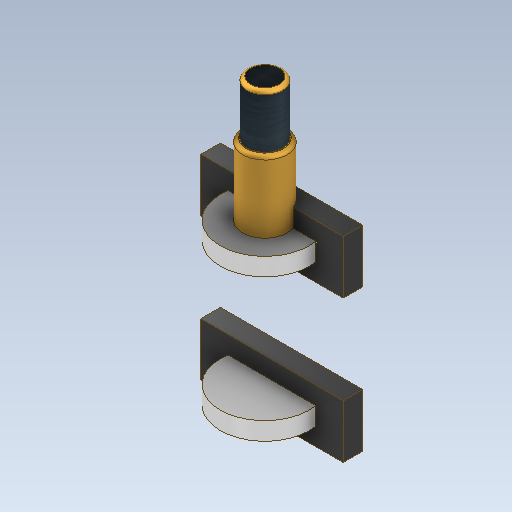
# Autodesk Inventor part: joint 2
Saved by Autodesk Inventor 2020 (Build 240168000, 168)
## iProperties
Created: 2020-07-11
Part Number: joint 2
Material: Aluminum 6061
Document SubType Name: Modeling
Designer: Vikki
Mass: 269.594 g
Surface Area: 274.025 cm^2
Volume: 99.8495 cm^3
Density: 2.7 g/cm^3
Appearance: Brass - Satin
Author: Vikki
Autodesk Inventor part; units mm, degrees
ref_plane "YZ Plane" through (0, 0, 0) normal (1, 0, 0) x (0, 1, 0)
ref_plane "XZ Plane" through (0, 0, 0) normal (0, 1, 0) x (-1, 0, 0)
ref_plane "XY Plane" through (0, 0, 0) normal (0, 0, 1) x (1, 0, 0)
ref_plane "Work Plane1" through (-25, -80, 5) normal (0, -1, 0) x (1, 0, 0)
ref_plane "Work Plane2" through (0, 0, 0) normal (0, 0, 1) x (1, 0, 0)
sketch "Sketch1" plane through (0, 0, 0) normal (0, 0, 1) x (1, 0, 0)
  line L0 (-65, -15) -> (15, -15)
  line L1 (15, -15) -> (15, 15)
  line L2 (15, 15) -> (-65, 15)
  line L3 (-65, 15) -> (-65, -15)
  line L4 (-65, -95) -> (15, -95)
  line L5 (15, -95) -> (15, -65)
  line L6 (15, -65) -> (-65, -65)
  line L7 (-65, -65) -> (-65, -95)
  line L8 (-46.7, 10) -> (-41.5, 10) projected
  arc A0 (-46.7, 10) -> (-46.9, 9.8) centre (-46.7, 9.8) ccw projected
  line L9 (-46.9, 8.2) -> (-46.9, 9.8) projected
  arc A1 (-46.9, 8.2) -> (-46.7, 8) centre (-46.7, 8.2) ccw projected
  line L10 (-43.8971, 8) -> (-46.7, 8) projected
  arc A2 (-43.7556, 7.6586) -> (-43.8971, 8) centre (-43.8971, 7.8) ccw projected
  line L11 (-47.3556, 4.0586) -> (-43.7556, 7.6586) projected
  arc A3 (-47.4971, 4) -> (-47.3556, 4.0586) centre (-47.4971, 4.2) ccw projected
  line L12 (-52.5029, 4) -> (-47.4971, 4) projected
  arc A4 (-52.6444, 4.0586) -> (-52.5029, 4) centre (-52.5029, 4.2) ccw projected
  line L13 (-56.2444, 7.6586) -> (-52.6444, 4.0586) projected
  arc A5 (-56.1029, 8) -> (-56.2444, 7.6586) centre (-56.1029, 7.8) ccw projected
  line L14 (-53.3, 8) -> (-56.1029, 8) projected
  arc A6 (-53.3, 8) -> (-53.1, 8.2) centre (-53.3, 8.2) ccw projected
  line L15 (-53.1, 9.8) -> (-53.1, 8.2) projected
  arc A7 (-53.1, 9.8) -> (-53.3, 10) centre (-53.3, 9.8) ccw projected
  line L16 (-58.5, 10) -> (-53.3, 10) projected
  arc A8 (-58.5, 10) -> (-60, 8.5) centre (-58.5, 8.5) ccw projected
  line L17 (-60, 3.3) -> (-60, 8.5) projected
  arc A9 (-60, 3.3) -> (-59.8, 3.1) centre (-59.8, 3.3) ccw projected
  line L18 (-58.2, 3.1) -> (-59.8, 3.1) projected
  arc A10 (-58.2, 3.1) -> (-58, 3.3) centre (-58.2, 3.3) ccw projected
  line L19 (-58, 6.1029) -> (-58, 3.3) projected
  arc A11 (-57.6586, 6.2444) -> (-58, 6.1029) centre (-57.8, 6.1029) ccw projected
  line L20 (-54.0586, 2.6444) -> (-57.6586, 6.2444) projected
  arc A12 (-54, 2.5029) -> (-54.0586, 2.6444) centre (-54.2, 2.5029) ccw projected
  line L21 (-54, -2.5029) -> (-54, 2.5029) projected
  arc A13 (-54.0586, -2.6444) -> (-54, -2.5029) centre (-54.2, -2.5029) ccw projected
  line L22 (-57.6586, -6.2444) -> (-54.0586, -2.6444) projected
  arc A14 (-58, -6.1029) -> (-57.6586, -6.2444) centre (-57.8, -6.1029) ccw projected
  line L23 (-58, -3.3) -> (-58, -6.1029) projected
  arc A15 (-58, -3.3) -> (-58.2, -3.1) centre (-58.2, -3.3) ccw projected
  line L24 (-59.8, -3.1) -> (-58.2, -3.1) projected
  arc A16 (-59.8, -3.1) -> (-60, -3.3) centre (-59.8, -3.3) ccw projected
  line L25 (-60, -8.5) -> (-60, -3.3) projected
  arc A17 (-60, -8.5) -> (-58.5, -10) centre (-58.5, -8.5) ccw projected
  line L26 (-53.3, -10) -> (-58.5, -10) projected
  arc A18 (-53.3, -10) -> (-53.1, -9.8) centre (-53.3, -9.8) ccw projected
  line L27 (-53.1, -8.2) -> (-53.1, -9.8) projected
  arc A19 (-53.1, -8.2) -> (-53.3, -8) centre (-53.3, -8.2) ccw projected
  line L28 (-56.1029, -8) -> (-53.3, -8) projected
  arc A20 (-56.2444, -7.6586) -> (-56.1029, -8) centre (-56.1029, -7.8) ccw projected
  line L29 (-52.6444, -4.0586) -> (-56.2444, -7.6586) projected
  arc A21 (-52.5029, -4) -> (-52.6444, -4.0586) centre (-52.5029, -4.2) ccw projected
  line L30 (-47.4971, -4) -> (-52.5029, -4) projected
  arc A22 (-47.3556, -4.0586) -> (-47.4971, -4) centre (-47.4971, -4.2) ccw projected
  line L31 (-43.7556, -7.6586) -> (-47.3556, -4.0586) projected
  arc A23 (-43.8971, -8) -> (-43.7556, -7.6586) centre (-43.8971, -7.8) ccw projected
  line L32 (-46.7, -8) -> (-43.8971, -8) projected
  arc A24 (-46.7, -8) -> (-46.9, -8.2) centre (-46.7, -8.2) ccw projected
  line L33 (-46.9, -9.8) -> (-46.9, -8.2) projected
  arc A25 (-46.9, -9.8) -> (-46.7, -10) centre (-46.7, -9.8) ccw projected
  line L34 (-41.5, -10) -> (-46.7, -10) projected
  arc A26 (-41.5, -10) -> (-40, -8.5) centre (-41.5, -8.5) ccw projected
  line L35 (-40, -3.3) -> (-40, -8.5) projected
  arc A27 (-40, -3.3) -> (-40.2, -3.1) centre (-40.2, -3.3) ccw projected
  line L36 (-41.8, -3.1) -> (-40.2, -3.1) projected
  arc A28 (-41.8, -3.1) -> (-42, -3.3) centre (-41.8, -3.3) ccw projected
  line L37 (-42, -6.1029) -> (-42, -3.3) projected
  arc A29 (-42.3414, -6.2444) -> (-42, -6.1029) centre (-42.2, -6.1029) ccw projected
  line L38 (-45.9414, -2.6444) -> (-42.3414, -6.2444) projected
  arc A30 (-46, -2.5029) -> (-45.9414, -2.6444) centre (-45.8, -2.5029) ccw projected
  line L39 (-46, 2.5029) -> (-46, -2.5029) projected
  arc A31 (-45.9414, 2.6444) -> (-46, 2.5029) centre (-45.8, 2.5029) ccw projected
  line L40 (-42.3414, 6.2444) -> (-45.9414, 2.6444) projected
  arc A32 (-42, 6.1029) -> (-42.3414, 6.2444) centre (-42.2, 6.1029) ccw projected
  line L41 (-42, 3.3) -> (-42, 6.1029) projected
  arc A33 (-42, 3.3) -> (-41.8, 3.1) centre (-41.8, 3.3) ccw projected
  line L42 (-40.2, 3.1) -> (-41.8, 3.1) projected
  arc A34 (-40.2, 3.1) -> (-40, 3.3) centre (-40.2, 3.3) ccw projected
  line L43 (-40, 8.5) -> (-40, 3.3) projected
  arc A35 (-40, 8.5) -> (-41.5, 10) centre (-41.5, 8.5) ccw projected
  circle A36 centre (-50, 0) radius 2 projected
  line L44 (3.3, 10) -> (8.5, 10) projected
  arc A37 (3.3, 10) -> (3.1, 9.8) centre (3.3, 9.8) ccw projected
  line L45 (3.1, 8.2) -> (3.1, 9.8) projected
  arc A38 (3.1, 8.2) -> (3.3, 8) centre (3.3, 8.2) ccw projected
  line L46 (6.1029, 8) -> (3.3, 8) projected
  arc A39 (6.2444, 7.6586) -> (6.1029, 8) centre (6.1029, 7.8) ccw projected
  line L47 (2.6444, 4.0586) -> (6.2444, 7.6586) projected
  arc A40 (2.5029, 4) -> (2.6444, 4.0586) centre (2.5029, 4.2) ccw projected
  line L48 (-2.5029, 4) -> (2.5029, 4) projected
  arc A41 (-2.6444, 4.0586) -> (-2.5029, 4) centre (-2.5029, 4.2) ccw projected
  line L49 (-6.2444, 7.6586) -> (-2.6444, 4.0586) projected
  arc A42 (-6.1029, 8) -> (-6.2444, 7.6586) centre (-6.1029, 7.8) ccw projected
  line L50 (-3.3, 8) -> (-6.1029, 8) projected
  arc A43 (-3.3, 8) -> (-3.1, 8.2) centre (-3.3, 8.2) ccw projected
  line L51 (-3.1, 9.8) -> (-3.1, 8.2) projected
  arc A44 (-3.1, 9.8) -> (-3.3, 10) centre (-3.3, 9.8) ccw projected
  line L52 (-8.5, 10) -> (-3.3, 10) projected
  arc A45 (-8.5, 10) -> (-10, 8.5) centre (-8.5, 8.5) ccw projected
  line L53 (-10, 3.3) -> (-10, 8.5) projected
  arc A46 (-10, 3.3) -> (-9.8, 3.1) centre (-9.8, 3.3) ccw projected
  line L54 (-8.2, 3.1) -> (-9.8, 3.1) projected
  arc A47 (-8.2, 3.1) -> (-8, 3.3) centre (-8.2, 3.3) ccw projected
  line L55 (-8, 6.1029) -> (-8, 3.3) projected
  arc A48 (-7.6586, 6.2444) -> (-8, 6.1029) centre (-7.8, 6.1029) ccw projected
  line L56 (-4.0586, 2.6444) -> (-7.6586, 6.2444) projected
  arc A49 (-4, 2.5029) -> (-4.0586, 2.6444) centre (-4.2, 2.5029) ccw projected
  line L57 (-4, -2.5029) -> (-4, 2.5029) projected
  arc A50 (-4.0586, -2.6444) -> (-4, -2.5029) centre (-4.2, -2.5029) ccw projected
  line L58 (-7.6586, -6.2444) -> (-4.0586, -2.6444) projected
  arc A51 (-8, -6.1029) -> (-7.6586, -6.2444) centre (-7.8, -6.1029) ccw projected
  line L59 (-8, -3.3) -> (-8, -6.1029) projected
  arc A52 (-8, -3.3) -> (-8.2, -3.1) centre (-8.2, -3.3) ccw projected
  line L60 (-9.8, -3.1) -> (-8.2, -3.1) projected
  arc A53 (-9.8, -3.1) -> (-10, -3.3) centre (-9.8, -3.3) ccw projected
  line L61 (-10, -8.5) -> (-10, -3.3) projected
  arc A54 (-10, -8.5) -> (-8.5, -10) centre (-8.5, -8.5) ccw projected
  line L62 (-3.3, -10) -> (-8.5, -10) projected
  arc A55 (-3.3, -10) -> (-3.1, -9.8) centre (-3.3, -9.8) ccw projected
  line L63 (-3.1, -8.2) -> (-3.1, -9.8) projected
  arc A56 (-3.1, -8.2) -> (-3.3, -8) centre (-3.3, -8.2) ccw projected
  line L64 (-6.1029, -8) -> (-3.3, -8) projected
  arc A57 (-6.2444, -7.6586) -> (-6.1029, -8) centre (-6.1029, -7.8) ccw projected
  line L65 (-2.6444, -4.0586) -> (-6.2444, -7.6586) projected
  arc A58 (-2.5029, -4) -> (-2.6444, -4.0586) centre (-2.5029, -4.2) ccw projected
  line L66 (2.5029, -4) -> (-2.5029, -4) projected
  arc A59 (2.6444, -4.0586) -> (2.5029, -4) centre (2.5029, -4.2) ccw projected
  line L67 (6.2444, -7.6586) -> (2.6444, -4.0586) projected
  arc A60 (6.1029, -8) -> (6.2444, -7.6586) centre (6.1029, -7.8) ccw projected
  line L68 (3.3, -8) -> (6.1029, -8) projected
  arc A61 (3.3, -8) -> (3.1, -8.2) centre (3.3, -8.2) ccw projected
  line L69 (3.1, -9.8) -> (3.1, -8.2) projected
  arc A62 (3.1, -9.8) -> (3.3, -10) centre (3.3, -9.8) ccw projected
  line L70 (8.5, -10) -> (3.3, -10) projected
  arc A63 (8.5, -10) -> (10, -8.5) centre (8.5, -8.5) ccw projected
  line L71 (10, -3.3) -> (10, -8.5) projected
  arc A64 (10, -3.3) -> (9.8, -3.1) centre (9.8, -3.3) ccw projected
  line L72 (8.2, -3.1) -> (9.8, -3.1) projected
  arc A65 (8.2, -3.1) -> (8, -3.3) centre (8.2, -3.3) ccw projected
  line L73 (8, -6.1029) -> (8, -3.3) projected
  arc A66 (7.6586, -6.2444) -> (8, -6.1029) centre (7.8, -6.1029) ccw projected
  line L74 (4.0586, -2.6444) -> (7.6586, -6.2444) projected
  arc A67 (4, -2.5029) -> (4.0586, -2.6444) centre (4.2, -2.5029) ccw projected
  line L75 (4, 2.5029) -> (4, -2.5029) projected
  arc A68 (4.0586, 2.6444) -> (4, 2.5029) centre (4.2, 2.5029) ccw projected
  line L76 (7.6586, 6.2444) -> (4.0586, 2.6444) projected
  arc A69 (8, 6.1029) -> (7.6586, 6.2444) centre (7.8, 6.1029) ccw projected
  line L77 (8, 3.3) -> (8, 6.1029) projected
  arc A70 (8, 3.3) -> (8.2, 3.1) centre (8.2, 3.3) ccw projected
  line L78 (9.8, 3.1) -> (8.2, 3.1) projected
  arc A71 (9.8, 3.1) -> (10, 3.3) centre (9.8, 3.3) ccw projected
  line L79 (10, 8.5) -> (10, 3.3) projected
  arc A72 (10, 8.5) -> (8.5, 10) centre (8.5, 8.5) ccw projected
  circle A73 centre (0, 0) radius 2 projected
  line L80 (-46.7, -70) -> (-41.5, -70) projected
  arc A74 (-46.7, -70) -> (-46.9, -70.2) centre (-46.7, -70.2) ccw projected
  line L81 (-46.9, -71.8) -> (-46.9, -70.2) projected
  arc A75 (-46.9, -71.8) -> (-46.7, -72) centre (-46.7, -71.8) ccw projected
  line L82 (-43.8971, -72) -> (-46.7, -72) projected
  arc A76 (-43.7556, -72.3414) -> (-43.8971, -72) centre (-43.8971, -72.2) ccw projected
  line L83 (-47.3556, -75.9414) -> (-43.7556, -72.3414) projected
  arc A77 (-47.4971, -76) -> (-47.3556, -75.9414) centre (-47.4971, -75.8) ccw projected
  line L84 (-52.5029, -76) -> (-47.4971, -76) projected
  arc A78 (-52.6444, -75.9414) -> (-52.5029, -76) centre (-52.5029, -75.8) ccw projected
  line L85 (-56.2444, -72.3414) -> (-52.6444, -75.9414) projected
  arc A79 (-56.1029, -72) -> (-56.2444, -72.3414) centre (-56.1029, -72.2) ccw projected
  line L86 (-53.3, -72) -> (-56.1029, -72) projected
  arc A80 (-53.3, -72) -> (-53.1, -71.8) centre (-53.3, -71.8) ccw projected
  line L87 (-53.1, -70.2) -> (-53.1, -71.8) projected
  arc A81 (-53.1, -70.2) -> (-53.3, -70) centre (-53.3, -70.2) ccw projected
  line L88 (-58.5, -70) -> (-53.3, -70) projected
  arc A82 (-58.5, -70) -> (-60, -71.5) centre (-58.5, -71.5) ccw projected
  line L89 (-60, -76.7) -> (-60, -71.5) projected
  arc A83 (-60, -76.7) -> (-59.8, -76.9) centre (-59.8, -76.7) ccw projected
  line L90 (-58.2, -76.9) -> (-59.8, -76.9) projected
  arc A84 (-58.2, -76.9) -> (-58, -76.7) centre (-58.2, -76.7) ccw projected
  line L91 (-58, -73.8971) -> (-58, -76.7) projected
  arc A85 (-57.6586, -73.7556) -> (-58, -73.8971) centre (-57.8, -73.8971) ccw projected
  line L92 (-54.0586, -77.3556) -> (-57.6586, -73.7556) projected
  arc A86 (-54, -77.4971) -> (-54.0586, -77.3556) centre (-54.2, -77.4971) ccw projected
  line L93 (-54, -82.5029) -> (-54, -77.4971) projected
  arc A87 (-54.0586, -82.6444) -> (-54, -82.5029) centre (-54.2, -82.5029) ccw projected
  line L94 (-57.6586, -86.2444) -> (-54.0586, -82.6444) projected
  arc A88 (-58, -86.1029) -> (-57.6586, -86.2444) centre (-57.8, -86.1029) ccw projected
  line L95 (-58, -83.3) -> (-58, -86.1029) projected
  arc A89 (-58, -83.3) -> (-58.2, -83.1) centre (-58.2, -83.3) ccw projected
  line L96 (-59.8, -83.1) -> (-58.2, -83.1) projected
  arc A90 (-59.8, -83.1) -> (-60, -83.3) centre (-59.8, -83.3) ccw projected
  line L97 (-60, -88.5) -> (-60, -83.3) projected
  arc A91 (-60, -88.5) -> (-58.5, -90) centre (-58.5, -88.5) ccw projected
  line L98 (-53.3, -90) -> (-58.5, -90) projected
  arc A92 (-53.3, -90) -> (-53.1, -89.8) centre (-53.3, -89.8) ccw projected
  line L99 (-53.1, -88.2) -> (-53.1, -89.8) projected
  arc A93 (-53.1, -88.2) -> (-53.3, -88) centre (-53.3, -88.2) ccw projected
  line L100 (-56.1029, -88) -> (-53.3, -88) projected
  arc A94 (-56.2444, -87.6586) -> (-56.1029, -88) centre (-56.1029, -87.8) ccw projected
  line L101 (-52.6444, -84.0586) -> (-56.2444, -87.6586) projected
  arc A95 (-52.5029, -84) -> (-52.6444, -84.0586) centre (-52.5029, -84.2) ccw projected
  line L102 (-47.4971, -84) -> (-52.5029, -84) projected
  arc A96 (-47.3556, -84.0586) -> (-47.4971, -84) centre (-47.4971, -84.2) ccw projected
  line L103 (-43.7556, -87.6586) -> (-47.3556, -84.0586) projected
  arc A97 (-43.8971, -88) -> (-43.7556, -87.6586) centre (-43.8971, -87.8) ccw projected
  line L104 (-46.7, -88) -> (-43.8971, -88) projected
  arc A98 (-46.7, -88) -> (-46.9, -88.2) centre (-46.7, -88.2) ccw projected
  line L105 (-46.9, -89.8) -> (-46.9, -88.2) projected
  arc A99 (-46.9, -89.8) -> (-46.7, -90) centre (-46.7, -89.8) ccw projected
  line L106 (-41.5, -90) -> (-46.7, -90) projected
  arc A100 (-41.5, -90) -> (-40, -88.5) centre (-41.5, -88.5) ccw projected
  line L107 (-40, -83.3) -> (-40, -88.5) projected
  arc A101 (-40, -83.3) -> (-40.2, -83.1) centre (-40.2, -83.3) ccw projected
  line L108 (-41.8, -83.1) -> (-40.2, -83.1) projected
  arc A102 (-41.8, -83.1) -> (-42, -83.3) centre (-41.8, -83.3) ccw projected
  line L109 (-42, -86.1029) -> (-42, -83.3) projected
  arc A103 (-42.3414, -86.2444) -> (-42, -86.1029) centre (-42.2, -86.1029) ccw projected
  line L110 (-45.9414, -82.6444) -> (-42.3414, -86.2444) projected
  arc A104 (-46, -82.5029) -> (-45.9414, -82.6444) centre (-45.8, -82.5029) ccw projected
  line L111 (-46, -77.4971) -> (-46, -82.5029) projected
  arc A105 (-45.9414, -77.3556) -> (-46, -77.4971) centre (-45.8, -77.4971) ccw projected
  line L112 (-42.3414, -73.7556) -> (-45.9414, -77.3556) projected
  arc A106 (-42, -73.8971) -> (-42.3414, -73.7556) centre (-42.2, -73.8971) ccw projected
  line L113 (-42, -76.7) -> (-42, -73.8971) projected
  arc A107 (-42, -76.7) -> (-41.8, -76.9) centre (-41.8, -76.7) ccw projected
  line L114 (-40.2, -76.9) -> (-41.8, -76.9) projected
  arc A108 (-40.2, -76.9) -> (-40, -76.7) centre (-40.2, -76.7) ccw projected
  line L115 (-40, -71.5) -> (-40, -76.7) projected
  arc A109 (-40, -71.5) -> (-41.5, -70) centre (-41.5, -71.5) ccw projected
  circle A110 centre (-50, -80) radius 2 projected
  line L116 (3.3, -70) -> (8.5, -70) projected
  arc A111 (3.3, -70) -> (3.1, -70.2) centre (3.3, -70.2) ccw projected
  line L117 (3.1, -71.8) -> (3.1, -70.2) projected
  arc A112 (3.1, -71.8) -> (3.3, -72) centre (3.3, -71.8) ccw projected
  line L118 (6.1029, -72) -> (3.3, -72) projected
  arc A113 (6.2444, -72.3414) -> (6.1029, -72) centre (6.1029, -72.2) ccw projected
  line L119 (2.6444, -75.9414) -> (6.2444, -72.3414) projected
  arc A114 (2.5029, -76) -> (2.6444, -75.9414) centre (2.5029, -75.8) ccw projected
  line L120 (-2.5029, -76) -> (2.5029, -76) projected
  arc A115 (-2.6444, -75.9414) -> (-2.5029, -76) centre (-2.5029, -75.8) ccw projected
  line L121 (-6.2444, -72.3414) -> (-2.6444, -75.9414) projected
  arc A116 (-6.1029, -72) -> (-6.2444, -72.3414) centre (-6.1029, -72.2) ccw projected
  line L122 (-3.3, -72) -> (-6.1029, -72) projected
  arc A117 (-3.3, -72) -> (-3.1, -71.8) centre (-3.3, -71.8) ccw projected
  line L123 (-3.1, -70.2) -> (-3.1, -71.8) projected
  arc A118 (-3.1, -70.2) -> (-3.3, -70) centre (-3.3, -70.2) ccw projected
  line L124 (-8.5, -70) -> (-3.3, -70) projected
  arc A119 (-8.5, -70) -> (-10, -71.5) centre (-8.5, -71.5) ccw projected
  line L125 (-10, -76.7) -> (-10, -71.5) projected
  arc A120 (-10, -76.7) -> (-9.8, -76.9) centre (-9.8, -76.7) ccw projected
  line L126 (-8.2, -76.9) -> (-9.8, -76.9) projected
  arc A121 (-8.2, -76.9) -> (-8, -76.7) centre (-8.2, -76.7) ccw projected
  line L127 (-8, -73.8971) -> (-8, -76.7) projected
  arc A122 (-7.6586, -73.7556) -> (-8, -73.8971) centre (-7.8, -73.8971) ccw projected
  line L128 (-4.0586, -77.3556) -> (-7.6586, -73.7556) projected
  arc A123 (-4, -77.4971) -> (-4.0586, -77.3556) centre (-4.2, -77.4971) ccw projected
  line L129 (-4, -82.5029) -> (-4, -77.4971) projected
  arc A124 (-4.0586, -82.6444) -> (-4, -82.5029) centre (-4.2, -82.5029) ccw projected
  line L130 (-7.6586, -86.2444) -> (-4.0586, -82.6444) projected
  arc A125 (-8, -86.1029) -> (-7.6586, -86.2444) centre (-7.8, -86.1029) ccw projected
  line L131 (-8, -83.3) -> (-8, -86.1029) projected
  arc A126 (-8, -83.3) -> (-8.2, -83.1) centre (-8.2, -83.3) ccw projected
  line L132 (-9.8, -83.1) -> (-8.2, -83.1) projected
  arc A127 (-9.8, -83.1) -> (-10, -83.3) centre (-9.8, -83.3) ccw projected
  line L133 (-10, -88.5) -> (-10, -83.3) projected
  arc A128 (-10, -88.5) -> (-8.5, -90) centre (-8.5, -88.5) ccw projected
  line L134 (-3.3, -90) -> (-8.5, -90) projected
  arc A129 (-3.3, -90) -> (-3.1, -89.8) centre (-3.3, -89.8) ccw projected
  line L135 (-3.1, -88.2) -> (-3.1, -89.8) projected
  arc A130 (-3.1, -88.2) -> (-3.3, -88) centre (-3.3, -88.2) ccw projected
  line L136 (-6.1029, -88) -> (-3.3, -88) projected
  arc A131 (-6.2444, -87.6586) -> (-6.1029, -88) centre (-6.1029, -87.8) ccw projected
  line L137 (-2.6444, -84.0586) -> (-6.2444, -87.6586) projected
  arc A132 (-2.5029, -84) -> (-2.6444, -84.0586) centre (-2.5029, -84.2) ccw projected
  line L138 (2.5029, -84) -> (-2.5029, -84) projected
  arc A133 (2.6444, -84.0586) -> (2.5029, -84) centre (2.5029, -84.2) ccw projected
  line L139 (6.2444, -87.6586) -> (2.6444, -84.0586) projected
  arc A134 (6.1029, -88) -> (6.2444, -87.6586) centre (6.1029, -87.8) ccw projected
  line L140 (3.3, -88) -> (6.1029, -88) projected
  arc A135 (3.3, -88) -> (3.1, -88.2) centre (3.3, -88.2) ccw projected
  line L141 (3.1, -89.8) -> (3.1, -88.2) projected
  arc A136 (3.1, -89.8) -> (3.3, -90) centre (3.3, -89.8) ccw projected
  line L142 (8.5, -90) -> (3.3, -90) projected
  arc A137 (8.5, -90) -> (10, -88.5) centre (8.5, -88.5) ccw projected
  line L143 (10, -83.3) -> (10, -88.5) projected
  arc A138 (10, -83.3) -> (9.8, -83.1) centre (9.8, -83.3) ccw projected
  line L144 (8.2, -83.1) -> (9.8, -83.1) projected
  arc A139 (8.2, -83.1) -> (8, -83.3) centre (8.2, -83.3) ccw projected
  line L145 (8, -86.1029) -> (8, -83.3) projected
  arc A140 (7.6586, -86.2444) -> (8, -86.1029) centre (7.8, -86.1029) ccw projected
  line L146 (4.0586, -82.6444) -> (7.6586, -86.2444) projected
  arc A141 (4, -82.5029) -> (4.0586, -82.6444) centre (4.2, -82.5029) ccw projected
  line L147 (4, -77.4971) -> (4, -82.5029) projected
  arc A142 (4.0586, -77.3556) -> (4, -77.4971) centre (4.2, -77.4971) ccw projected
  line L148 (7.6586, -73.7556) -> (4.0586, -77.3556) projected
  arc A143 (8, -73.8971) -> (7.6586, -73.7556) centre (7.8, -73.8971) ccw projected
  line L149 (8, -76.7) -> (8, -73.8971) projected
  arc A144 (8, -76.7) -> (8.2, -76.9) centre (8.2, -76.7) ccw projected
  line L150 (9.8, -76.9) -> (8.2, -76.9) projected
  arc A145 (9.8, -76.9) -> (10, -76.7) centre (9.8, -76.7) ccw projected
  line L151 (10, -71.5) -> (10, -76.7) projected
  arc A146 (10, -71.5) -> (8.5, -70) centre (8.5, -71.5) ccw projected
  circle A147 centre (0, -80) radius 2 projected
  point P0 (0, 0)
  dimension "d0" = 5
  dimension "d1" = 5
  dimension "d2" = 5
  dimension "d3" = 5
  dimension "d4" = 5
  dimension "d5" = 5
  dimension "d6" = 5
  dimension "d7" = 5
  constraints: 16 end point, 4 parallel, 2 horizontal, 2 perpendicular
  measures "d0" distance between parallel lines of L2 L16
  measures "d1" distance between parallel lines of L0 L34
  measures "d2" distance between parallel lines of L3 L17
  measures "d3" distance between parallel lines of L79 L1
  measures "d4" distance between parallel lines of L7 L89
  measures "d5" distance between parallel lines of L143 L5
  measures "d6" distance between parallel lines of L4 L142
  measures "d7" distance between parallel lines of L6 L124
extrude "Extrusion1" add sketch "Sketch1" against normal blind 10 contours L3 L2 L1 L0 | L7 L6 L5 L4
sketch "Sketch2" plane through (0, 0, 0) normal (0, 0, 1) x (1, 0, 0)
  line L0 (-46.7, -70) -> (-41.5, -70) projected
  arc A0 (-46.7, -70) -> (-46.9, -70.2) centre (-46.7, -70.2) ccw projected
  line L1 (-46.9, -71.8) -> (-46.9, -70.2) projected
  arc A1 (-46.9, -71.8) -> (-46.7, -72) centre (-46.7, -71.8) ccw projected
  line L2 (-43.8971, -72) -> (-46.7, -72) projected
  arc A2 (-43.7556, -72.3414) -> (-43.8971, -72) centre (-43.8971, -72.2) ccw projected
  line L3 (-47.3556, -75.9414) -> (-43.7556, -72.3414) projected
  arc A3 (-47.4971, -76) -> (-47.3556, -75.9414) centre (-47.4971, -75.8) ccw projected
  line L4 (-52.5029, -76) -> (-47.4971, -76) projected
  arc A4 (-52.6444, -75.9414) -> (-52.5029, -76) centre (-52.5029, -75.8) ccw projected
  line L5 (-56.2444, -72.3414) -> (-52.6444, -75.9414) projected
  arc A5 (-56.1029, -72) -> (-56.2444, -72.3414) centre (-56.1029, -72.2) ccw projected
  line L6 (-53.3, -72) -> (-56.1029, -72) projected
  arc A6 (-53.3, -72) -> (-53.1, -71.8) centre (-53.3, -71.8) ccw projected
  line L7 (-53.1, -70.2) -> (-53.1, -71.8) projected
  arc A7 (-53.1, -70.2) -> (-53.3, -70) centre (-53.3, -70.2) ccw projected
  line L8 (-58.5, -70) -> (-53.3, -70) projected
  arc A8 (-58.5, -70) -> (-60, -71.5) centre (-58.5, -71.5) ccw projected
  line L9 (-60, -76.7) -> (-60, -71.5) projected
  arc A9 (-60, -76.7) -> (-59.8, -76.9) centre (-59.8, -76.7) ccw projected
  line L10 (-58.2, -76.9) -> (-59.8, -76.9) projected
  arc A10 (-58.2, -76.9) -> (-58, -76.7) centre (-58.2, -76.7) ccw projected
  line L11 (-58, -73.8971) -> (-58, -76.7) projected
  arc A11 (-57.6586, -73.7556) -> (-58, -73.8971) centre (-57.8, -73.8971) ccw projected
  line L12 (-54.0586, -77.3556) -> (-57.6586, -73.7556) projected
  arc A12 (-54, -77.4971) -> (-54.0586, -77.3556) centre (-54.2, -77.4971) ccw projected
  line L13 (-54, -82.5029) -> (-54, -77.4971) projected
  arc A13 (-54.0586, -82.6444) -> (-54, -82.5029) centre (-54.2, -82.5029) ccw projected
  line L14 (-57.6586, -86.2444) -> (-54.0586, -82.6444) projected
  arc A14 (-58, -86.1029) -> (-57.6586, -86.2444) centre (-57.8, -86.1029) ccw projected
  line L15 (-58, -83.3) -> (-58, -86.1029) projected
  arc A15 (-58, -83.3) -> (-58.2, -83.1) centre (-58.2, -83.3) ccw projected
  line L16 (-59.8, -83.1) -> (-58.2, -83.1) projected
  arc A16 (-59.8, -83.1) -> (-60, -83.3) centre (-59.8, -83.3) ccw projected
  line L17 (-60, -88.5) -> (-60, -83.3) projected
  arc A17 (-60, -88.5) -> (-58.5, -90) centre (-58.5, -88.5) ccw projected
  line L18 (-53.3, -90) -> (-58.5, -90) projected
  arc A18 (-53.3, -90) -> (-53.1, -89.8) centre (-53.3, -89.8) ccw projected
  line L19 (-53.1, -88.2) -> (-53.1, -89.8) projected
  arc A19 (-53.1, -88.2) -> (-53.3, -88) centre (-53.3, -88.2) ccw projected
  line L20 (-56.1029, -88) -> (-53.3, -88) projected
  arc A20 (-56.2444, -87.6586) -> (-56.1029, -88) centre (-56.1029, -87.8) ccw projected
  line L21 (-52.6444, -84.0586) -> (-56.2444, -87.6586) projected
  arc A21 (-52.5029, -84) -> (-52.6444, -84.0586) centre (-52.5029, -84.2) ccw projected
  line L22 (-47.4971, -84) -> (-52.5029, -84) projected
  arc A22 (-47.3556, -84.0586) -> (-47.4971, -84) centre (-47.4971, -84.2) ccw projected
  line L23 (-43.7556, -87.6586) -> (-47.3556, -84.0586) projected
  arc A23 (-43.8971, -88) -> (-43.7556, -87.6586) centre (-43.8971, -87.8) ccw projected
  line L24 (-46.7, -88) -> (-43.8971, -88) projected
  arc A24 (-46.7, -88) -> (-46.9, -88.2) centre (-46.7, -88.2) ccw projected
  line L25 (-46.9, -89.8) -> (-46.9, -88.2) projected
  arc A25 (-46.9, -89.8) -> (-46.7, -90) centre (-46.7, -89.8) ccw projected
  line L26 (-41.5, -90) -> (-46.7, -90) projected
  arc A26 (-41.5, -90) -> (-40, -88.5) centre (-41.5, -88.5) ccw projected
  line L27 (-40, -83.3) -> (-40, -88.5) projected
  arc A27 (-40, -83.3) -> (-40.2, -83.1) centre (-40.2, -83.3) ccw projected
  line L28 (-41.8, -83.1) -> (-40.2, -83.1) projected
  arc A28 (-41.8, -83.1) -> (-42, -83.3) centre (-41.8, -83.3) ccw projected
  line L29 (-42, -86.1029) -> (-42, -83.3) projected
  arc A29 (-42.3414, -86.2444) -> (-42, -86.1029) centre (-42.2, -86.1029) ccw projected
  line L30 (-45.9414, -82.6444) -> (-42.3414, -86.2444) projected
  arc A30 (-46, -82.5029) -> (-45.9414, -82.6444) centre (-45.8, -82.5029) ccw projected
  line L31 (-46, -77.4971) -> (-46, -82.5029) projected
  arc A31 (-45.9414, -77.3556) -> (-46, -77.4971) centre (-45.8, -77.4971) ccw projected
  line L32 (-42.3414, -73.7556) -> (-45.9414, -77.3556) projected
  arc A32 (-42, -73.8971) -> (-42.3414, -73.7556) centre (-42.2, -73.8971) ccw projected
  line L33 (-42, -76.7) -> (-42, -73.8971) projected
  arc A33 (-42, -76.7) -> (-41.8, -76.9) centre (-41.8, -76.7) ccw projected
  line L34 (-40.2, -76.9) -> (-41.8, -76.9) projected
  arc A34 (-40.2, -76.9) -> (-40, -76.7) centre (-40.2, -76.7) ccw projected
  line L35 (-40, -71.5) -> (-40, -76.7) projected
  arc A35 (-40, -71.5) -> (-41.5, -70) centre (-41.5, -71.5) ccw projected
  circle A36 centre (-50, -80) radius 2 projected
  line L36 (3.3, -70) -> (8.5, -70) projected
  arc A37 (3.3, -70) -> (3.1, -70.2) centre (3.3, -70.2) ccw projected
  line L37 (3.1, -71.8) -> (3.1, -70.2) projected
  arc A38 (3.1, -71.8) -> (3.3, -72) centre (3.3, -71.8) ccw projected
  line L38 (6.1029, -72) -> (3.3, -72) projected
  arc A39 (6.2444, -72.3414) -> (6.1029, -72) centre (6.1029, -72.2) ccw projected
  line L39 (2.6444, -75.9414) -> (6.2444, -72.3414) projected
  arc A40 (2.5029, -76) -> (2.6444, -75.9414) centre (2.5029, -75.8) ccw projected
  line L40 (-2.5029, -76) -> (2.5029, -76) projected
  arc A41 (-2.6444, -75.9414) -> (-2.5029, -76) centre (-2.5029, -75.8) ccw projected
  line L41 (-6.2444, -72.3414) -> (-2.6444, -75.9414) projected
  arc A42 (-6.1029, -72) -> (-6.2444, -72.3414) centre (-6.1029, -72.2) ccw projected
  line L42 (-3.3, -72) -> (-6.1029, -72) projected
  arc A43 (-3.3, -72) -> (-3.1, -71.8) centre (-3.3, -71.8) ccw projected
  line L43 (-3.1, -70.2) -> (-3.1, -71.8) projected
  arc A44 (-3.1, -70.2) -> (-3.3, -70) centre (-3.3, -70.2) ccw projected
  line L44 (-8.5, -70) -> (-3.3, -70) projected
  arc A45 (-8.5, -70) -> (-10, -71.5) centre (-8.5, -71.5) ccw projected
  line L45 (-10, -76.7) -> (-10, -71.5) projected
  arc A46 (-10, -76.7) -> (-9.8, -76.9) centre (-9.8, -76.7) ccw projected
  line L46 (-8.2, -76.9) -> (-9.8, -76.9) projected
  arc A47 (-8.2, -76.9) -> (-8, -76.7) centre (-8.2, -76.7) ccw projected
  line L47 (-8, -73.8971) -> (-8, -76.7) projected
  arc A48 (-7.6586, -73.7556) -> (-8, -73.8971) centre (-7.8, -73.8971) ccw projected
  line L48 (-4.0586, -77.3556) -> (-7.6586, -73.7556) projected
  arc A49 (-4, -77.4971) -> (-4.0586, -77.3556) centre (-4.2, -77.4971) ccw projected
  line L49 (-4, -82.5029) -> (-4, -77.4971) projected
  arc A50 (-4.0586, -82.6444) -> (-4, -82.5029) centre (-4.2, -82.5029) ccw projected
  line L50 (-7.6586, -86.2444) -> (-4.0586, -82.6444) projected
  arc A51 (-8, -86.1029) -> (-7.6586, -86.2444) centre (-7.8, -86.1029) ccw projected
  line L51 (-8, -83.3) -> (-8, -86.1029) projected
  arc A52 (-8, -83.3) -> (-8.2, -83.1) centre (-8.2, -83.3) ccw projected
  line L52 (-9.8, -83.1) -> (-8.2, -83.1) projected
  arc A53 (-9.8, -83.1) -> (-10, -83.3) centre (-9.8, -83.3) ccw projected
  line L53 (-10, -88.5) -> (-10, -83.3) projected
  arc A54 (-10, -88.5) -> (-8.5, -90) centre (-8.5, -88.5) ccw projected
  line L54 (-3.3, -90) -> (-8.5, -90) projected
  arc A55 (-3.3, -90) -> (-3.1, -89.8) centre (-3.3, -89.8) ccw projected
  line L55 (-3.1, -88.2) -> (-3.1, -89.8) projected
  arc A56 (-3.1, -88.2) -> (-3.3, -88) centre (-3.3, -88.2) ccw projected
  line L56 (-6.1029, -88) -> (-3.3, -88) projected
  arc A57 (-6.2444, -87.6586) -> (-6.1029, -88) centre (-6.1029, -87.8) ccw projected
  line L57 (-2.6444, -84.0586) -> (-6.2444, -87.6586) projected
  arc A58 (-2.5029, -84) -> (-2.6444, -84.0586) centre (-2.5029, -84.2) ccw projected
  line L58 (2.5029, -84) -> (-2.5029, -84) projected
  arc A59 (2.6444, -84.0586) -> (2.5029, -84) centre (2.5029, -84.2) ccw projected
  line L59 (6.2444, -87.6586) -> (2.6444, -84.0586) projected
  arc A60 (6.1029, -88) -> (6.2444, -87.6586) centre (6.1029, -87.8) ccw projected
  line L60 (3.3, -88) -> (6.1029, -88) projected
  arc A61 (3.3, -88) -> (3.1, -88.2) centre (3.3, -88.2) ccw projected
  line L61 (3.1, -89.8) -> (3.1, -88.2) projected
  arc A62 (3.1, -89.8) -> (3.3, -90) centre (3.3, -89.8) ccw projected
  line L62 (8.5, -90) -> (3.3, -90) projected
  arc A63 (8.5, -90) -> (10, -88.5) centre (8.5, -88.5) ccw projected
  line L63 (10, -83.3) -> (10, -88.5) projected
  arc A64 (10, -83.3) -> (9.8, -83.1) centre (9.8, -83.3) ccw projected
  line L64 (8.2, -83.1) -> (9.8, -83.1) projected
  arc A65 (8.2, -83.1) -> (8, -83.3) centre (8.2, -83.3) ccw projected
  line L65 (8, -86.1029) -> (8, -83.3) projected
  arc A66 (7.6586, -86.2444) -> (8, -86.1029) centre (7.8, -86.1029) ccw projected
  line L66 (4.0586, -82.6444) -> (7.6586, -86.2444) projected
  arc A67 (4, -82.5029) -> (4.0586, -82.6444) centre (4.2, -82.5029) ccw projected
  line L67 (4, -77.4971) -> (4, -82.5029) projected
  arc A68 (4.0586, -77.3556) -> (4, -77.4971) centre (4.2, -77.4971) ccw projected
  line L68 (7.6586, -73.7556) -> (4.0586, -77.3556) projected
  arc A69 (8, -73.8971) -> (7.6586, -73.7556) centre (7.8, -73.8971) ccw projected
  line L69 (8, -76.7) -> (8, -73.8971) projected
  arc A70 (8, -76.7) -> (8.2, -76.9) centre (8.2, -76.7) ccw projected
  line L70 (9.8, -76.9) -> (8.2, -76.9) projected
  arc A71 (9.8, -76.9) -> (10, -76.7) centre (9.8, -76.7) ccw projected
  line L71 (10, -71.5) -> (10, -76.7) projected
  arc A72 (10, -71.5) -> (8.5, -70) centre (8.5, -71.5) ccw projected
  circle A73 centre (0, -80) radius 2 projected
  line L72 (3.3, 10) -> (8.5, 10) projected
  arc A74 (3.3, 10) -> (3.1, 9.8) centre (3.3, 9.8) ccw projected
  line L73 (3.1, 8.2) -> (3.1, 9.8) projected
  arc A75 (3.1, 8.2) -> (3.3, 8) centre (3.3, 8.2) ccw projected
  line L74 (6.1029, 8) -> (3.3, 8) projected
  arc A76 (6.2444, 7.6586) -> (6.1029, 8) centre (6.1029, 7.8) ccw projected
  line L75 (2.6444, 4.0586) -> (6.2444, 7.6586) projected
  arc A77 (2.5029, 4) -> (2.6444, 4.0586) centre (2.5029, 4.2) ccw projected
  line L76 (-2.5029, 4) -> (2.5029, 4) projected
  arc A78 (-2.6444, 4.0586) -> (-2.5029, 4) centre (-2.5029, 4.2) ccw projected
  line L77 (-6.2444, 7.6586) -> (-2.6444, 4.0586) projected
  arc A79 (-6.1029, 8) -> (-6.2444, 7.6586) centre (-6.1029, 7.8) ccw projected
  line L78 (-3.3, 8) -> (-6.1029, 8) projected
  arc A80 (-3.3, 8) -> (-3.1, 8.2) centre (-3.3, 8.2) ccw projected
  line L79 (-3.1, 9.8) -> (-3.1, 8.2) projected
  arc A81 (-3.1, 9.8) -> (-3.3, 10) centre (-3.3, 9.8) ccw projected
  line L80 (-8.5, 10) -> (-3.3, 10) projected
  arc A82 (-8.5, 10) -> (-10, 8.5) centre (-8.5, 8.5) ccw projected
  line L81 (-10, 3.3) -> (-10, 8.5) projected
  arc A83 (-10, 3.3) -> (-9.8, 3.1) centre (-9.8, 3.3) ccw projected
  line L82 (-8.2, 3.1) -> (-9.8, 3.1) projected
  arc A84 (-8.2, 3.1) -> (-8, 3.3) centre (-8.2, 3.3) ccw projected
  line L83 (-8, 6.1029) -> (-8, 3.3) projected
  arc A85 (-7.6586, 6.2444) -> (-8, 6.1029) centre (-7.8, 6.1029) ccw projected
  line L84 (-4.0586, 2.6444) -> (-7.6586, 6.2444) projected
  arc A86 (-4, 2.5029) -> (-4.0586, 2.6444) centre (-4.2, 2.5029) ccw projected
  line L85 (-4, -2.5029) -> (-4, 2.5029) projected
  arc A87 (-4.0586, -2.6444) -> (-4, -2.5029) centre (-4.2, -2.5029) ccw projected
  line L86 (-7.6586, -6.2444) -> (-4.0586, -2.6444) projected
  arc A88 (-8, -6.1029) -> (-7.6586, -6.2444) centre (-7.8, -6.1029) ccw projected
  line L87 (-8, -3.3) -> (-8, -6.1029) projected
  arc A89 (-8, -3.3) -> (-8.2, -3.1) centre (-8.2, -3.3) ccw projected
  line L88 (-9.8, -3.1) -> (-8.2, -3.1) projected
  arc A90 (-9.8, -3.1) -> (-10, -3.3) centre (-9.8, -3.3) ccw projected
  line L89 (-10, -8.5) -> (-10, -3.3) projected
  arc A91 (-10, -8.5) -> (-8.5, -10) centre (-8.5, -8.5) ccw projected
  line L90 (-3.3, -10) -> (-8.5, -10) projected
  arc A92 (-3.3, -10) -> (-3.1, -9.8) centre (-3.3, -9.8) ccw projected
  line L91 (-3.1, -8.2) -> (-3.1, -9.8) projected
  arc A93 (-3.1, -8.2) -> (-3.3, -8) centre (-3.3, -8.2) ccw projected
  line L92 (-6.1029, -8) -> (-3.3, -8) projected
  arc A94 (-6.2444, -7.6586) -> (-6.1029, -8) centre (-6.1029, -7.8) ccw projected
  line L93 (-2.6444, -4.0586) -> (-6.2444, -7.6586) projected
  arc A95 (-2.5029, -4) -> (-2.6444, -4.0586) centre (-2.5029, -4.2) ccw projected
  line L94 (2.5029, -4) -> (-2.5029, -4) projected
  arc A96 (2.6444, -4.0586) -> (2.5029, -4) centre (2.5029, -4.2) ccw projected
  line L95 (6.2444, -7.6586) -> (2.6444, -4.0586) projected
  arc A97 (6.1029, -8) -> (6.2444, -7.6586) centre (6.1029, -7.8) ccw projected
  line L96 (3.3, -8) -> (6.1029, -8) projected
  arc A98 (3.3, -8) -> (3.1, -8.2) centre (3.3, -8.2) ccw projected
  line L97 (3.1, -9.8) -> (3.1, -8.2) projected
  arc A99 (3.1, -9.8) -> (3.3, -10) centre (3.3, -9.8) ccw projected
  line L98 (8.5, -10) -> (3.3, -10) projected
  arc A100 (8.5, -10) -> (10, -8.5) centre (8.5, -8.5) ccw projected
  line L99 (10, -3.3) -> (10, -8.5) projected
  arc A101 (10, -3.3) -> (9.8, -3.1) centre (9.8, -3.3) ccw projected
  line L100 (8.2, -3.1) -> (9.8, -3.1) projected
  arc A102 (8.2, -3.1) -> (8, -3.3) centre (8.2, -3.3) ccw projected
  line L101 (8, -6.1029) -> (8, -3.3) projected
  arc A103 (7.6586, -6.2444) -> (8, -6.1029) centre (7.8, -6.1029) ccw projected
  line L102 (4.0586, -2.6444) -> (7.6586, -6.2444) projected
  arc A104 (4, -2.5029) -> (4.0586, -2.6444) centre (4.2, -2.5029) ccw projected
  line L103 (4, 2.5029) -> (4, -2.5029) projected
  arc A105 (4.0586, 2.6444) -> (4, 2.5029) centre (4.2, 2.5029) ccw projected
  line L104 (7.6586, 6.2444) -> (4.0586, 2.6444) projected
  arc A106 (8, 6.1029) -> (7.6586, 6.2444) centre (7.8, 6.1029) ccw projected
  line L105 (8, 3.3) -> (8, 6.1029) projected
  arc A107 (8, 3.3) -> (8.2, 3.1) centre (8.2, 3.3) ccw projected
  line L106 (9.8, 3.1) -> (8.2, 3.1) projected
  arc A108 (9.8, 3.1) -> (10, 3.3) centre (9.8, 3.3) ccw projected
  line L107 (10, 8.5) -> (10, 3.3) projected
  arc A109 (10, 8.5) -> (8.5, 10) centre (8.5, 8.5) ccw projected
  circle A110 centre (0, 0) radius 2 projected
  line L108 (-46.7, 10) -> (-41.5, 10) projected
  arc A111 (-46.7, 10) -> (-46.9, 9.8) centre (-46.7, 9.8) ccw projected
  line L109 (-46.9, 8.2) -> (-46.9, 9.8) projected
  arc A112 (-46.9, 8.2) -> (-46.7, 8) centre (-46.7, 8.2) ccw projected
  line L110 (-43.8971, 8) -> (-46.7, 8) projected
  arc A113 (-43.7556, 7.6586) -> (-43.8971, 8) centre (-43.8971, 7.8) ccw projected
  line L111 (-47.3556, 4.0586) -> (-43.7556, 7.6586) projected
  arc A114 (-47.4971, 4) -> (-47.3556, 4.0586) centre (-47.4971, 4.2) ccw projected
  line L112 (-52.5029, 4) -> (-47.4971, 4) projected
  arc A115 (-52.6444, 4.0586) -> (-52.5029, 4) centre (-52.5029, 4.2) ccw projected
  line L113 (-56.2444, 7.6586) -> (-52.6444, 4.0586) projected
  arc A116 (-56.1029, 8) -> (-56.2444, 7.6586) centre (-56.1029, 7.8) ccw projected
  line L114 (-53.3, 8) -> (-56.1029, 8) projected
  arc A117 (-53.3, 8) -> (-53.1, 8.2) centre (-53.3, 8.2) ccw projected
  line L115 (-53.1, 9.8) -> (-53.1, 8.2) projected
  arc A118 (-53.1, 9.8) -> (-53.3, 10) centre (-53.3, 9.8) ccw projected
  line L116 (-58.5, 10) -> (-53.3, 10) projected
  arc A119 (-58.5, 10) -> (-60, 8.5) centre (-58.5, 8.5) ccw projected
  line L117 (-60, 3.3) -> (-60, 8.5) projected
  arc A120 (-60, 3.3) -> (-59.8, 3.1) centre (-59.8, 3.3) ccw projected
  line L118 (-58.2, 3.1) -> (-59.8, 3.1) projected
  arc A121 (-58.2, 3.1) -> (-58, 3.3) centre (-58.2, 3.3) ccw projected
  line L119 (-58, 6.1029) -> (-58, 3.3) projected
  arc A122 (-57.6586, 6.2444) -> (-58, 6.1029) centre (-57.8, 6.1029) ccw projected
  line L120 (-54.0586, 2.6444) -> (-57.6586, 6.2444) projected
  arc A123 (-54, 2.5029) -> (-54.0586, 2.6444) centre (-54.2, 2.5029) ccw projected
  line L121 (-54, -2.5029) -> (-54, 2.5029) projected
  arc A124 (-54.0586, -2.6444) -> (-54, -2.5029) centre (-54.2, -2.5029) ccw projected
  line L122 (-57.6586, -6.2444) -> (-54.0586, -2.6444) projected
  arc A125 (-58, -6.1029) -> (-57.6586, -6.2444) centre (-57.8, -6.1029) ccw projected
  line L123 (-58, -3.3) -> (-58, -6.1029) projected
  arc A126 (-58, -3.3) -> (-58.2, -3.1) centre (-58.2, -3.3) ccw projected
  line L124 (-59.8, -3.1) -> (-58.2, -3.1) projected
  arc A127 (-59.8, -3.1) -> (-60, -3.3) centre (-59.8, -3.3) ccw projected
  line L125 (-60, -8.5) -> (-60, -3.3) projected
  arc A128 (-60, -8.5) -> (-58.5, -10) centre (-58.5, -8.5) ccw projected
  line L126 (-53.3, -10) -> (-58.5, -10) projected
  arc A129 (-53.3, -10) -> (-53.1, -9.8) centre (-53.3, -9.8) ccw projected
  line L127 (-53.1, -8.2) -> (-53.1, -9.8) projected
  arc A130 (-53.1, -8.2) -> (-53.3, -8) centre (-53.3, -8.2) ccw projected
  line L128 (-56.1029, -8) -> (-53.3, -8) projected
  arc A131 (-56.2444, -7.6586) -> (-56.1029, -8) centre (-56.1029, -7.8) ccw projected
  line L129 (-52.6444, -4.0586) -> (-56.2444, -7.6586) projected
  arc A132 (-52.5029, -4) -> (-52.6444, -4.0586) centre (-52.5029, -4.2) ccw projected
  line L130 (-47.4971, -4) -> (-52.5029, -4) projected
  arc A133 (-47.3556, -4.0586) -> (-47.4971, -4) centre (-47.4971, -4.2) ccw projected
  line L131 (-43.7556, -7.6586) -> (-47.3556, -4.0586) projected
  arc A134 (-43.8971, -8) -> (-43.7556, -7.6586) centre (-43.8971, -7.8) ccw projected
  line L132 (-46.7, -8) -> (-43.8971, -8) projected
  arc A135 (-46.7, -8) -> (-46.9, -8.2) centre (-46.7, -8.2) ccw projected
  line L133 (-46.9, -9.8) -> (-46.9, -8.2) projected
  arc A136 (-46.9, -9.8) -> (-46.7, -10) centre (-46.7, -9.8) ccw projected
  line L134 (-41.5, -10) -> (-46.7, -10) projected
  arc A137 (-41.5, -10) -> (-40, -8.5) centre (-41.5, -8.5) ccw projected
  line L135 (-40, -3.3) -> (-40, -8.5) projected
  arc A138 (-40, -3.3) -> (-40.2, -3.1) centre (-40.2, -3.3) ccw projected
  line L136 (-41.8, -3.1) -> (-40.2, -3.1) projected
  arc A139 (-41.8, -3.1) -> (-42, -3.3) centre (-41.8, -3.3) ccw projected
  line L137 (-42, -6.1029) -> (-42, -3.3) projected
  arc A140 (-42.3414, -6.2444) -> (-42, -6.1029) centre (-42.2, -6.1029) ccw projected
  line L138 (-45.9414, -2.6444) -> (-42.3414, -6.2444) projected
  arc A141 (-46, -2.5029) -> (-45.9414, -2.6444) centre (-45.8, -2.5029) ccw projected
  line L139 (-46, 2.5029) -> (-46, -2.5029) projected
  arc A142 (-45.9414, 2.6444) -> (-46, 2.5029) centre (-45.8, 2.5029) ccw projected
  line L140 (-42.3414, 6.2444) -> (-45.9414, 2.6444) projected
  arc A143 (-42, 6.1029) -> (-42.3414, 6.2444) centre (-42.2, 6.1029) ccw projected
  line L141 (-42, 3.3) -> (-42, 6.1029) projected
  arc A144 (-42, 3.3) -> (-41.8, 3.1) centre (-41.8, 3.3) ccw projected
  line L142 (-40.2, 3.1) -> (-41.8, 3.1) projected
  arc A145 (-40.2, 3.1) -> (-40, 3.3) centre (-40.2, 3.3) ccw projected
  line L143 (-40, 8.5) -> (-40, 3.3) projected
  arc A146 (-40, 8.5) -> (-41.5, 10) centre (-41.5, 8.5) ccw projected
  circle A147 centre (-50, 0) radius 2 projected
  line L144 (-65, -65) -> (-65, -95) projected
  line L145 (15, -65) -> (-65, -65) projected
  line L146 (-65, -95) -> (15, -95) projected
  line L147 (15, -95) -> (15, -65) projected
  line L148 (15, -15) -> (15, 15) projected
  line L149 (15, 15) -> (-65, 15) projected
  line L150 (-65, -15) -> (15, -15) projected
  line L151 (-65, 15) -> (-65, -15) projected
  point P0 (0, 0)
extrude "Extrusion2" add sketch "Sketch2" against normal blind 5 contours L0 A35 L35 A34 L34 A33 L33 A32 L32 A31 L31 A30 L30 A29 L29 A28 L28 A27 L27 A26 L26 A25 L25 A24 L24 A23 L23 A22 L22 A21 L21 A20 L20 A19 L19 A18 L18 A17 L17 A16 L16 A15 L15 A14 L14 A13 L13 A12 L12 A11 L11 A10 L10 A9 L9 A8 L8 A7 L7 A6 L6 A5 L5 A4 L4 A3 L3 A2 L2 A1 L1 A0 | A36 | L36 A72 L71 A71 L70 A70 L69 A69 L68 A68 L67 A67 L66 A66 L65 A65 L64 A64 L63 A63 L62 A62 L61 A61 L60 A60 L59 A59 L58 A58 L57 A57 L56 A56 L55 A55 L54 A54 L53 A53 L52 A52 L51 A51 L50 A50 L49 A49 L48 A48 L47 A47 L46 A46 L45 A45 L44 A44 L43 A43 L42 A42 L41 A41 L40 A40 L39 A39 L38 A38 L37 A37 | A73 | L72 A109 L107 A108 L106 A107 L105 A106 L104 A105 L103 A104 L102 A103 L101 A102 L100 A101 L99 A100 L98 A99 L97 A98 L96 A97 L95 A96 L94 A95 L93 A94 L92 A93 L91 A92 L90 A91 L89 A90 L88 A89 L87 A88 L86 A87 L85 A86 L84 A85 L83 A84 L82 A83 L81 A82 L80 A81 L79 A80 L78 A79 L77 A78 L76 A77 L75 A76 L74 A75 L73 A74 | A110 | L108 A146 L143 A145 L142 A144 L141 A143 L140 A142 L139 A141 L138 A140 L137 A139 L136 A138 L135 A137 L134 A136 L133 A135 L132 A134 L131 A133 L130 A132 L129 A131 L128 A130 L127 A129 L126 A128 L125 A127 L124 A126 L123 A125 L122 A124 L121 A123 L120 A122 L119 A121 L118 A120 L117 A119 L116 A118 L115 A117 L114 A116 L113 A115 L112 A114 L111 A113 L110 A112 L109 A111 | A147
sketch "Sketch3" plane through (0, 0, 0) normal (0, 0, 1) x (1, 0, 0)
  line L0 (15, -95) -> (15, -65) projected
  line L1 (15, -65) -> (-65, -65) projected
  line L2 (-65, -65) -> (-65, -95) projected
  line L3 (-65, -95) -> (15, -95) projected
  line L4 (-65, 15) -> (-65, -15) projected
  line L5 (-65, -15) -> (15, -15) projected
  line L6 (15, -15) -> (15, 15) projected
  line L7 (15, 15) -> (-65, 15) projected
  point P0 (0, 0)
extrude "Extrusion3" add sketch "Sketch3" along normal blind 1
sketch "Sketch4" plane through (-25, -80, 5) normal (0, -1, 0) x (1, 0, 0)
  arc A0 (25, 0) -> (-25, 0) centre (0, 0) ccw projected
  circle A1 centre (0, 0) radius 25
  line L0 (-40, -4) -> (40, -4) projected
  point P0 (25, -5)
  point P1 (-24.6779, -4)
  point P2 (24.6779, -4)
  point P3 (25, 0)
  point P4 (-25, 0)
  dimension "d14" = 0
  constraints: 1 centre point, 1 coincident
  measures "d14" radial gap between concentric circles of A0 A1
extrude "Extrusion4" add sketch "Sketch4" along normal mid plane 10 contours A1 L0 A0
pattern_linear "Rectangular Pattern1" count 2 spacing 80 along (0, 1, 0) of "Extrusion4"
sketch "Sketch5" plane through (-25, 5, 5) normal (0, 1, 0) x (1, 0, 0)
  point P0 (25, 5)
sketch "Sketch6" plane through (-25, 5, 5) normal (0, 1, 0) x (1, 0, 0)
  circle A0 centre (0, 0) radius 12.5
  point P0 (25, 5)
  dimension "d20" = 25
  constraints: 1 centre point
  measures "d20" diameter of A0
extrude "Extrusion5" add sketch "Sketch6" along normal blind 40
sketch "Sketch7" plane through (-25, 45, 5) normal (0, 1, 0) x (1, 0, 0)
  circle A0 centre (0, 0) radius 5 projected
  circle A1 centre (0, 0) radius 10
  point P0 (25, 5)
  dimension "d23" = 20
  constraints: 1 centre point, 1 coincident
  measures "d23" diameter of A1
extrude "Extrusion6" add sketch "Sketch7" along normal blind 30 contours A0 | A1
fillet "Fillet1" radius 2 2 edges at (-37.5, 45, 5) (-35, 75, 5)
body "Solid1"
